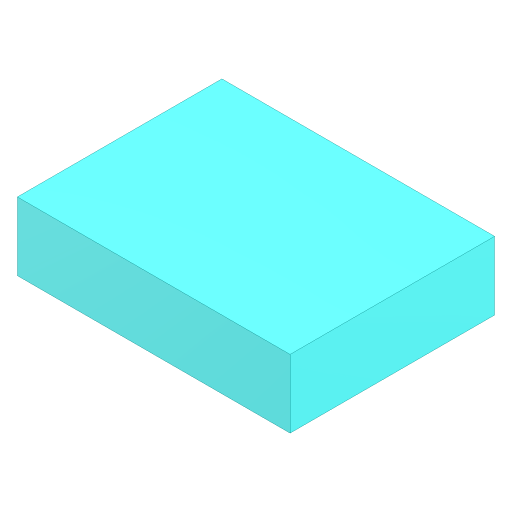
# Autodesk Inventor part: support_ladder
Saved by Autodesk Inventor 2024 (Build 280153000, 153)
## iProperties
Created: 2024-06-06
Part Number: support_ladder
Material: 一般
Document SubType Name: Modeling
Designer: admin
Density: 1 g/cm^3
Appearance: 平滑 - 灰白色
Author: admin
Autodesk Inventor part; units mm, degrees
ref_plane "YZ Plane" through (0, 0, 0) normal (1, 0, 0) x (0, 1, 0)
ref_plane "XZ Plane" through (0, 0, 0) normal (0, 1, 0) x (-1, 0, 0)
ref_plane "XY Plane" through (0, 0, 0) normal (0, 0, 1) x (1, 0, 0)
sketch "草圖3" plane through (0, 0, 0) normal (0, 1, 0) x (-1, 0, 0)
  line L0 (0, 0) -> (80, 0)
  line L1 (80, 0) -> (80, -60)
  line L2 (80, -60) -> (0, -60)
  line L3 (0, -60) -> (0, 0)
  dimension "d32" = 60
  dimension "d33" = 80
  constraints: 8 end point, 2 parallel, 1 horizontal, 1 perpendicular
  measures "d32" distance of L0.end L1.end
  measures "d33" distance of L1.end L2.end
extrude "擠出4" add sketch "草圖3" along normal blind 20
equation "\"d11\" = 1.6"
equation "\"d12\" = 11.6"
equation "\"d24\" = 1.6"
equation "\"d25\" = 11.6"
